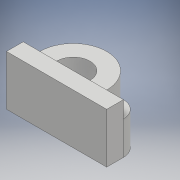
# Autodesk Inventor part: 4
Saved by Autodesk Inventor 2017 (Build 210142000, 142)
## iProperties
Part Number: 4
Material: 一般
Document SubType Name: Modeling
Designer: Brian
Density: 1 g/cm^3
Appearance: 預設
Author: Brian
Autodesk Inventor part; units mm, degrees
ref_plane "YZ Plane" through (0, 0, 0) normal (1, 0, 0) x (0, 1, 0)
ref_plane "XZ Plane" through (0, 0, 0) normal (0, 1, 0) x (-1, 0, 0)
ref_plane "XY Plane" through (0, 0, 0) normal (0, 0, 1) x (1, 0, 0)
sketch "草圖1" plane through (0, 0, 0) normal (0, 0, 1) x (1, 0, 0)
  line L0 (0, 0) -> (60, 0)
  line L1 (60, 0) -> (60, 20)
  line L2 (60, 20) -> (0, 20)
  line L3 (0, 20) -> (0, 0)
  line L4 (0, 20) -> (40, 20)
  line L5 (40, 20) -> (40, 40)
  line L6 (40, 40) -> (0, 40)
  line L7 (0, 40) -> (0, 20)
  dimension "d0" = 20
  dimension "d1" = 20
  dimension "d2" = 60
  dimension "d3" = 40
  constraints: 16 end point, 4 parallel, 2 horizontal, 2 perpendicular
  measures "d0" distance of L6.end L2.end
  measures "d1" distance of L2.end L0.start
  measures "d2" distance of L0.start L0.end
  measures "d3" distance of L5.end L6.end
extrude "擠出1" add sketch "草圖1" along normal blind 20
fillet "圓角1" radius 20 2 edges at (40, 40, 10) (0, 40, 10)
fillet "圓角2" radius 10 1 edges at (60, 20, 10)
sketch "草圖2" plane through (0, 0, 20) normal (0, 0, 1) x (1, 0, 0)
  line L0 (60, 0) -> (60, 10) projected
  line L1 (0, 20) -> (0, 0) projected
  line L2 (60, 10) -> (0, 10)
  line L3 (0, 10) -> (0, 0)
  line L4 (0, 0) -> (60, 0)
  line L5 (60, 0) -> (60, 10)
  constraints: 8 end point, 2 parallel, 1 horizontal, 1 perpendicular
extrude "擠出2" add sketch "草圖2" along normal blind 10
sketch "草圖3" plane through (0, 0, 20) normal (0, 0, 1) x (1, 0, 0)
  arc A0 (40, 20) -> (0, 20) centre (20, 20) ccw projected
  circle A1 centre (20, 20) radius 10
  line L0 (0, 10) -> (60, 10) projected
  point P0 (0, 0)
  constraints: 1 centre point, 1 coincident, 1 tangent
extrude "擠出3" cut sketch "草圖3" against normal through all
